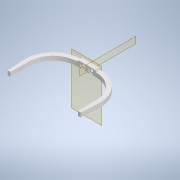
# Autodesk Inventor part: leg
Saved by Autodesk Inventor 2020 (Build 240168000, 168)
## iProperties
Created: 2019-05-08
Part Number: leg
Material: Generic
Document SubType Name: Modeling
Designer: erwin
Density: 1 g/cm^3
Appearance: Default
Author: erwin
Autodesk Inventor part; units mm, degrees
ref_plane "YZ Plane" through (0, 0, 0) normal (1, 0, 0) x (0, 1, 0)
ref_plane "XZ Plane" through (0, 0, 0) normal (0, 1, 0) x (-1, 0, 0)
ref_plane "XY Plane" through (0, 0, 0) normal (0, 0, 1) x (1, 0, 0)
ref_plane "Work Plane1" through (0, 0, 0) normal (0, 0, 1) x (1, 0, 0)
sketch "Sketch1" plane through (0, 0, 0) normal (0, 0, 1) x (1, 0, 0)
  circle A0 centre (10.2273, -23.9687) radius 0.75 projected
  circle A1 centre (0.7, 24) radius 0.75 projected
  circle A2 centre (10.2, 24) radius 0.75 projected
  circle A3 centre (0.7, -24) radius 0.75 projected
  arc A4 (-14, 7) -> (-16, 5) centre (-14, 5) ccw projected
  line L0 (-16, -15) -> (-16, 5) projected
  arc A5 (-16, -15) -> (-14, -17) centre (-14, -15) ccw projected
  line L1 (-8, -17) -> (-14, -17) projected
  arc A6 (-6, -19) -> (-8, -17) centre (-8, -19) ccw projected
  line L2 (-6, -25.5) -> (-6, -19) projected
  arc A7 (-6, -25.5) -> (-4, -27.5) centre (-4, -25.5) ccw projected
  line L3 (14, -27.5) -> (-4, -27.5) projected
  arc A8 (14, -27.5) -> (16, -25.5) centre (14, -25.5) ccw projected
  line L4 (16, -20.5) -> (16, -25.5) projected
  line L5 (-4, -20.5) -> (16, -20.5) projected
  line L6 (-4, -15) -> (-4, -20.5) projected
  line L7 (-14, -15) -> (-4, -15) projected
  line L8 (-14, 5) -> (-14, -15) projected
  line L9 (-4, 5) -> (-14, 5) projected
  line L10 (-4, 20.5) -> (-4, 5) projected
  line L11 (16, 20.5) -> (-4, 20.5) projected
  line L12 (16, 25.5) -> (16, 20.5) projected
  arc A9 (16, 25.5) -> (14, 27.5) centre (14, 25.5) ccw projected
  line L13 (-4, 27.5) -> (14, 27.5) projected
  arc A10 (-4, 27.5) -> (-6, 25.5) centre (-4, 25.5) ccw projected
  line L14 (-6, 9) -> (-6, 25.5) projected
  arc A11 (-8, 7) -> (-6, 9) centre (-8, 9) ccw projected
  line L15 (-14, 7) -> (-8, 7) projected
  line L16 (-4, 20.5) -> (-6, 20.5)
  point P0 (0, 0)
  constraints: 2 end point, 1 perpendicular, 1 point on line
extrude "Extrusion1" add sketch "Sketch1" along normal blind 5 contours L14 A10 L13 A9 L12 L11 L16
sketch "Sketch2" plane through (0, 0, 5) normal (0, 0, 1) x (1, 0, 0)
  circle A0 centre (0.7, 24) radius 0.75 projected
  circle A1 centre (10.2, 24) radius 0.75 projected
  point P0 (0, 0)
  constraints: 2 coincident
hole "Hole1" at (0.7, 24, 5) at (10.2, 24, 5) direction (0, 0, -1) diameter 3 end through all counterbore diameter 6.5 counterbore depth 1
sketch "Sketch4" plane through (-6, 20.5, 0) normal (0, -1, 0) x (1, 0, 0)
  line L0 (0, 0) -> (22, 0) projected
  line L1 (11.75, -1) -> (10.25, -1) construction
  line L2 (10.25, -1) -> (10.25, 1) construction
  line L3 (10.25, 1) -> (11.75, 1) construction
  line L4 (11.75, 1) -> (11.75, -1) construction
  line L5 (11.75, -1) -> (10.25, 1) construction
  line L6 (10.25, -1) -> (11.75, 1) construction
  line L7 (10.25, 1) -> (11.75, 1)
  line L8 (11.75, 1) -> (11.75, 0)
  line L9 (11.75, 0) -> (10.25, 0)
  line L10 (10.25, 0) -> (10.25, 1)
  point P0 (6, 0)
  point P1 (11, 0)
  dimension "d9" = 1.5
  dimension "d10" = 2
  constraints: 20 end point, 4 midpoint, 4 parallel, 2 horizontal, 2 perpendicular
  measures "d9" distance of L2.end L3.end
  measures "d10" distance of L1.end L2.end
extrude "Extrusion2" cut sketch "Sketch4" against normal through all
draft "FaceDraft1" angle 5 pull direction (0, -1, 0) faces at (5.25, 22.8333, 1) fixed edges at (5, 20.5, 1)
sketch "Sketch5" plane through (-6, 20.5, 5) normal (0, -1, 0) x (1, 0, 0)
  arc A0 (-33.2285, 30.645) -> (0, -5) centre (0, 28.3104) ccw
  line L0 (2, 0) -> (0, 0) projected
  arc A1 (-28.3785, 27.7601) -> (0, 0) centre (0, 28.3854) ccw
  line L1 (-33.2285, 30.645) -> (-31.8686, 50)
  line L2 (-31.8686, 50) -> (-28.8686, 50)
  line L3 (-28.8686, 50) -> (-28.3785, 27.7601)
  line L4 (0, 0) -> (22, 0) projected
  line L5 (0, -5) -> (10.25, -5) projected
  line L6 (0, -5) -> (0, 0) projected
  line L7 (0, -5) -> (0, 0)
  dimension "d15" = 50
  dimension "d16" = 3
  constraints: 8 end point, 4 point on circle, 4 tangent, 2 centre point, 1 collinear, 1 horizontal
  measures "d15" distance between parallel lines of L2 L4
  measures "d16" distance of L1.end L2.end
ref_plane "Work Plane2" through (5, 20.5, 0) normal (1, 0, 0) x (0, 0, -1)
extrude "Extrusion3" add sketch "Sketch5" against normal blind 5
mirror "Mirror1" about plane through (5, 20.5, 0) normal (1, 0, 0) of "Extrusion3"
body "Solid1"
